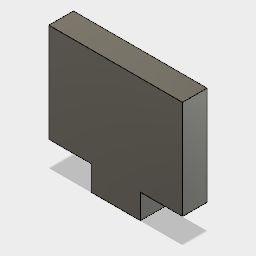
servo_guide3 v1 (Autodesk Fusion 360 design; units mm, degrees)
Autodesk Fusion 360 part; units mm, degrees
sketch "スケッチ1" plane through (0, 0, 0) normal (0, 0, 1) x (1, 0, 0)
  line L0 (173.9056, -200.0792) -> (173.9056, -202.5793)
  line L1 (183.1559, -190.0791) -> (169.639, -190.0791)
  line L2 (169.639, -200.0792) -> (173.9056, -200.0792)
  line L3 (178.9056, -202.5793) -> (178.9056, -200.0792)
  line L4 (178.9056, -200.0792) -> (183.1559, -200.0792)
  line L5 (169.639, -190.0791) -> (169.639, -200.0792)
  line L6 (173.9056, -202.5793) -> (178.9056, -202.5793)
  line L7 (183.1559, -200.0792) -> (183.1559, -190.0791)
extrude "押し出し1" add sketch "スケッチ1" along normal blind 2.5
